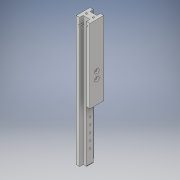
# Autodesk Inventor part: bACKBeamSplit
Saved by Autodesk Inventor 2019 (Build 230136000, 136)
## iProperties
Created: 2019-09-28
Part Number: bACKBeamSplit
Material: Generic
Document SubType Name: Modeling
Designer: james
Density: 1 g/cm^3
Appearance: Default
Author: james
Autodesk Inventor part; units mm, degrees
ref_plane "YZ Plane" through (0, 0, 0) normal (1, 0, 0) x (0, 1, 0)
ref_plane "XZ Plane" through (0, 0, 0) normal (0, 1, 0) x (-1, 0, 0)
ref_plane "XY Plane" through (0, 0, 0) normal (0, 0, 1) x (1, 0, 0)
sketch "Sketch1" plane through (0, 0, 0) normal (0, 1, 0) x (-1, 0, 0)
  line L0 (16.1925, 35.7868) -> (-9.2075, 35.7868)
  line L1 (-9.2075, 35.7868) -> (-9.2075, 10.3868)
  line L2 (-9.2075, 10.3868) -> (16.1925, 10.3868)
  line L3 (16.1925, 10.3868) -> (16.1925, 35.7868)
  point P0 (0, 0)
  dimension "d0" = 25.4
  dimension "d1" = 25.4
  constraints: 8 end point, 2 parallel, 1 horizontal, 1 perpendicular
  measures "d0" distance of L0.start L0.end
  measures "d1" distance of L0.end L1.end
extrude "Extrusion1" add sketch "Sketch1" along normal blind 368.3
sketch "Sketch2" plane through (0, 368.3, 0) normal (0, 1, 0) x (1, 0, 0)
  line L0 (-9.8425, -16.7368) -> (2.8575, -16.7368)
  line L1 (2.8575, -16.7368) -> (2.8575, -1.003)
  line L2 (2.8575, -1.003) -> (-9.8425, -1.003)
  line L3 (-9.8425, -1.003) -> (-9.8425, -16.7368)
  line L4 (9.2075, -35.7868) -> (9.2075, -10.3868) projected
  line L5 (-16.1925, -10.3868) -> (-16.1925, -35.7868) projected
  line L6 (9.2075, -10.3868) -> (-16.1925, -10.3868) projected
  point P0 (0, 0)
  dimension "d4" = 6.35
  dimension "d5" = 6.35
  dimension "d6" = 6.35
  constraints: 8 end point, 2 parallel, 1 horizontal, 1 perpendicular
  measures "d4" distance between parallel lines of L1 L4
  measures "d5" distance between parallel lines of L5 L3
  measures "d6" distance between parallel lines of L0 L6
extrude "Extrusion2" cut sketch "Sketch2" against normal blind 508
sketch "Sketch4" plane through (0, 368.3, 0) normal (0, 1, 0) x (1, 0, 0)
  line L0 (-9.8425, -29.4368) -> (2.8575, -29.4368)
  line L1 (2.8575, -29.4368) -> (2.8575, -45.8861)
  line L2 (2.8575, -45.8861) -> (-9.8425, -45.8861)
  line L3 (-9.8425, -45.8861) -> (-9.8425, -29.4368)
  line L4 (-16.1925, -10.3868) -> (-16.1925, -35.7868) projected
  line L5 (9.2075, -35.7868) -> (9.2075, -10.3868) projected
  line L6 (-16.1925, -35.7868) -> (9.2075, -35.7868) projected
  point P0 (0, 0)
  dimension "d20" = 6.35
  dimension "d21" = 6.35
  dimension "d22" = 6.35
  constraints: 8 end point, 2 parallel, 1 horizontal, 1 perpendicular
  measures "d20" distance between parallel lines of L3 L4
  measures "d21" distance between parallel lines of L5 L1
  measures "d22" distance between parallel lines of L6 L0
extrude "Extrusion3" cut sketch "Sketch4" against normal blind 508
sketch "Sketch5" plane through (9.2075, 0, 10.3868) normal (0, 0, -1) x (-1, 0, 0)
  line L0 (0, 0) -> (6.35, 0) projected
  line L1 (0, 0) -> (0, 368.3) projected
  line L2 (25.4, 0) -> (25.4, 368.3) projected
  line L3 (19.05, 0) -> (25.4, 0) projected
  point P0 (9.2075, 0)
  point P1 (19.05, 6.35)
  point P2 (6.35, 12.7)
  dimension "d25" = 12.7
  dimension "d27" = 6.35
  dimension "d28" = 6.35
  dimension "d60" = 19.05
  measures "d25" distance from line of L0 point (6.35, 12.7)
  measures "d27" distance from line of L2 point (19.05, 6.35)
  measures "d28" distance from line of L3 point (19.05, 6.35)
  measures "d60" distance from line of point (6.35, 12.7) L2
hole "Hole2" at (-9.8425, 6.35, 10.3868) at (2.8575, 12.7, 10.3868) direction (0, 0, 1) diameter 3.175 end through all
sketch "Sketch6" plane through (-16.1925, 0, 10.3868) normal (0, 0, -1) x (-1, 0, 0)
  line L0 (-6.35, 368.3) -> (-6.35, 7.9375) projected
  line L1 (-25.4, 368.3) -> (-19.05, 368.3) projected
  line L2 (-25.4, 0) -> (-25.4, 368.3) projected
  line L3 (-6.35, 368.3) -> (0, 368.3) projected
  line L4 (0, 0) -> (0, 368.3) projected
  point P0 (-16.1925, 0)
  point P1 (-19.05, 361.95)
  point P2 (-6.35, 355.6)
  dimension "d36" = 6.35
  dimension "d38" = 12.7
  dimension "d58" = 6.35
  dimension "d59" = 19.05
  constraints: 1 point on line
  measures "d36" distance from line of point (-19.05, 361.95) L1
  measures "d38" distance from line of L3 point (-6.35, 355.6)
  measures "d58" distance from line of L4 point (-6.35, 355.6)
  measures "d59" distance from line of point (-19.05, 361.95) L4
hole "Hole3" at (2.8575, 361.95, 10.3868) at (-9.8425, 355.6, 10.3868) direction (0, 0, 1) diameter 3.175 end through all
sketch "Sketch7" plane through (0, 0, 0) normal (0, -1, 0) x (1, 0, 0)
  line L0 (2.8575, 35.7868) -> (9.2075, 35.7868) projected
  line L1 (9.2075, 35.7868) -> (9.2075, 10.3868) projected
  line L2 (-16.1925, 10.3868) -> (-16.1925, 35.7868) projected
  line L3 (-16.1925, 35.7868) -> (-9.8425, 35.7868) projected
  point P0 (0, 0)
  point P1 (-9.8425, 23.0868)
  point P2 (2.8575, 23.0868)
  dimension "d47" = 12.7
  dimension "d48" = 6.35
  dimension "d49" = 6.35
  dimension "d50" = 12.7
  measures "d47" distance from line of L0 point (2.857, 23.087)
  measures "d48" distance from line of L1 point (2.857, 23.087)
  measures "d49" distance from line of L2 point (-9.843, 23.087)
  measures "d50" distance from line of L3 point (-9.843, 23.087)
hole "Hole4" at (-9.8425, 0, 23.0868) at (2.8575, 0, 23.0868) direction (0, 1, 0) diameter 3.175 end through all
sketch "Sketch8" plane through (-16.1925, 0, 35.7868) normal (0, 0, 1) x (1, 0, 0)
  line L0 (0, 0) -> (6.35, 0) projected
  line L1 (12.7, 231.775) -> (12.7, 130.175)
  line L2 (25.4, 0) -> (25.4, 368.3) projected
  line L3 (12.7, 231.775) -> (25.4, 231.775)
  line L4 (25.4, 231.775) -> (25.4, 156.0421)
  line L5 (25.4, 0) -> (25.4, 368.3) projected
  line L6 (12.7, 130.175) -> (-23.2246, 130.175)
  line L7 (25.4, 156.0421) -> (58.6697, 156.0421)
  line L8 (58.6697, 156.0421) -> (58.6697, -29.9503)
  line L9 (58.6697, -29.9503) -> (-23.2246, -29.1025)
  line L10 (-23.2246, -29.1025) -> (-23.2246, 130.175)
  line L11 (6.35, 368.3) -> (19.05, 368.3) projected
  point P0 (16.1925, 0)
  dimension "d62" = 12.7
  dimension "d110" = 101.6
  dimension "d111" = 136.525
  constraints: 16 end point, 3 horizontal, 2 point on line, 1 parallel, 1 perpendicular, 1 vertical
  measures "d62" distance between parallel lines of L1 L2
  measures "d110" distance of L1.start L1.end
  measures "d111" distance between parallel lines of L11 L3
extrude "Extrusion4" cut sketch "Sketch8" against normal blind 50.8
sketch "Sketch9" plane through (-16.1925, 368.3, 35.7868) normal (0, 0, 1) x (1, 0, 0)
  line L0 (12.6492, -136.4742) -> (52.9271, -136.4742)
  line L1 (52.9271, -136.4742) -> (52.9271, -241.0236)
  line L2 (52.9271, -241.0236) -> (12.6492, -241.0236)
  line L3 (12.6492, -241.0236) -> (12.6492, -136.4742)
  line L4 (12.7, -238.125) -> (12.7, -136.525) projected
  line L5 (19.05, -136.525) -> (25.4, -136.525) projected
  point P0 (16.1925, -368.3)
  dimension "d67" = 0.0508
  dimension "d68" = 0.0508
  constraints: 8 end point, 2 parallel, 1 horizontal, 1 perpendicular
  measures "d67" distance between parallel lines of L3 L4
  measures "d68" distance between parallel lines of L5 L0
extrude "Extrusion5" cut sketch "Sketch9" against normal blind 50.8
sketch "Sketch10" plane through (-16.1925, 368.3, 10.3868) normal (-1, 0, 0) x (0, 0, 1)
  line L0 (25.4, -238.125) -> (25.4, 0) projected
  line L1 (0, -238.125) -> (25.4, -238.125) projected
  point P0 (-10.3868, -368.3)
  point P1 (12.7, -161.925)
  point P2 (12.7, -187.325)
  point P3 (12.7, -174.625)
  point P4 (12.7, -212.725)
  point P5 (12.7, -200.025)
  dimension "d71" = 12.7
  dimension "d72" = 12.7
  dimension "d73" = 12.7
  dimension "d74" = 12.7
  dimension "d76" = 12.7
  dimension "d77" = 25.4
  dimension "d78" = 12.7
  dimension "d79" = 12.7
  dimension "d80" = 12.7
  dimension "d112" = 12.7
  measures "d71" distance from line of L0 point (12.7, -174.625)
  measures "d72" distance from line of L0 point (12.7, -212.725)
  measures "d73" distance from line of L0 point (12.7, -187.325)
  measures "d74" distance from line of L0 point (12.7, -161.925)
  measures "d76" distance of point (12.7, -174.625) point (12.7, -161.925)
  measures "d77" distance from line of L1 point (12.7, -212.725)
  measures "d78" distance of point (12.7, -187.325) point (12.7, -174.625)
  measures "d79" distance from line of L0 point (12.7, -200.025)
  measures "d80" distance of point (12.7, -187.325) point (12.7, -200.025)
  measures "d112" distance of point (12.7, -212.725) point (12.7, -200.025)
hole "Hole5" at (-16.1925, 206.375, 23.0868) at (-16.1925, 180.975, 23.0868) at (-16.1925, 193.675, 23.0868) at (-16.1925, 155.575, 23.0868) at (-16.1925, 168.275, 23.0868) direction (1, 0, 0) diameter 2.794 end through all countersink diameter 7.0866 countersink angle 82
sketch "Sketch11" plane through (-16.1925, 130.175, 35.7868) normal (0, -1, 0) x (1, 0, 0)
  circle A0 centre (6.35, -12.7) radius 1.5875 projected
  circle A1 centre (6.35, -12.7) radius 3.3147
  circle A2 centre (19.05, -12.7) radius 1.5875 projected
  point P0 (16.1925, -35.7868)
  dimension "d88" = 6.6294
  constraints: 1 centre point, 1 coincident
  measures "d88" diameter of A1
extrude "Extrusion6" cut sketch "Sketch11" against normal blind 19.304 contours A1
sketch "Sketch12" plane through (-3.5433, 231.8258, 16.7368) normal (0, -1, 0) x (1, 0, 0)
  circle A0 centre (6.4008, 6.35) radius 1.5875 projected
  circle A1 centre (6.4008, 6.35) radius 3.3147
  point P0 (3.5433, -16.7368)
  dimension "d92" = 6.6294
  constraints: 1 centre point, 1 coincident
  measures "d92" diameter of A1
extrude "Extrusion7" cut sketch "Sketch12" against normal blind 27.94
sketch "Sketch13" plane through (9.2075, 368.3, 35.7868) normal (1, 0, 0) x (0, 0, -1)
  line L0 (0, 0) -> (25.4, 0) projected
  line L1 (0, -136.4742) -> (0, 0) projected
  point P0 (35.7868, -368.3)
  point P1 (12.7, -82.55)
  point P2 (12.7, -95.25)
  dimension "d95" = 82.55
  dimension "d96" = 12.7
  dimension "d97" = 12.7
  dimension "d98" = 12.7
  measures "d95" distance from line of point (12.7, -82.55) L0
  measures "d96" distance from line of L1 point (12.7, -82.55)
  measures "d97" distance from line of L1 point (12.7, -95.25)
  measures "d98" distance of point (12.7, -95.25) point (12.7, -82.55)
hole "Hole6" at (9.2075, 285.75, 23.0868) at (9.2075, 273.05, 23.0868) direction (-1, 0, 0) diameter 4.4958 end through all countersink diameter 8.4328 countersink angle 82 clearance for "Flat Head Machine Screw (82)" size "#8" standard "Ansi Unified Screw Threads"
sketch "Sketch15" plane through (2.8575, 368.3, 35.7868) normal (0, 0, 1) x (1, 0, 0)
  line L0 (15.3531, -136.2837) -> (-6.5913, -136.2837)
  line L1 (-6.5913, -136.2837) -> (-6.5913, -237.4977)
  line L2 (-6.5913, -237.4977) -> (15.3531, -237.4977)
  line L3 (15.3531, -237.4977) -> (15.3531, -136.2837)
  line L4 (-6.4008, -238.125) -> (-6.4008, -136.4742) projected
  line L5 (-6.4008, -136.4742) -> (0, -136.4742) projected
  line L6 (0, -136.4742) -> (6.35, -136.4742) projected
  line L7 (6.35, -136.4742) -> (6.35, 0) projected
  line L8 (0, 0) -> (6.35, 0) projected
  line L9 (0, 0) -> (0, -4.7625) projected
  arc A0 (0, -7.9375) -> (0, -4.7625) centre (0, -6.35) ccw projected
  line L10 (0, -7.9375) -> (0, -136.4742) projected
  point P0 (-2.8575, -368.3)
  dimension "d106" = 0.1905
  dimension "d107" = 0.1905
  constraints: 8 end point, 2 parallel, 1 horizontal, 1 perpendicular
  measures "d106" distance between parallel lines of L6 L0
  measures "d107" distance between parallel lines of L4 L1
extrude "Extrusion8" cut sketch "Sketch15" against normal blind 50.8 contours L3 L2 L4 L5 L6 L7 L0 | L7 L6 L10 L0 | L10 L5 L4 L2 L1 L0
body "Solid1"
